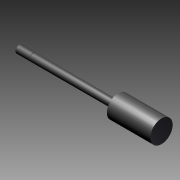
# Autodesk Inventor part: 0420_rod
Saved by Autodesk Inventor 2012 (Build 160160000, 160)
## iProperties
Category: PARTsolutions
Company: BIMBA
Created: 2013-01-19
Part Number: 0420_rod
Material: Default
Catalog Web Link: www.cadenas.de
Description: Standard Air Cylinder_rod-Original Line - Standard Air Cylinders
Vendor: BIMBA
Document SubType Name: Modeling
Designer: William
Manufacturer: BIMBA
Density: 1 g/cm^3
Mass: 13.5965 g
Surface Area: 45.5733 cm^2
Volume: 13.5965 cm^3
PSOL_IDENT_0: {\\10.0.0.242\data_v9\23d-libs\bimba\bimba\bimba_imperial\bimba_full_line\original_line_cylinders\st
PSOL_IDENT_1: andard_air_cylinders\rod.prj},270 {VTYP=3D},{NB=0420_rod},{LINA=0420_rod},{NN=Standard Air Cylinder_
PSOL_IDENT_2: rod},{DATE=11.09.2012 07:37:40},{GEOMDATE=06.09.2012 09:06:00},{VERSION=},{LINEID=50},{LINESUBID=-1}
PSOL_IDENT_3: ,{WBVAR=STROKE,ACTING,MNT,DER,NR,BM,CO,M,EE,EEL,K,Q,Y,F,G,T,B,H,SER,SR,NT,W,E,HL,ST,STP,PRC,PB,COLOR
PSOL_IDENT_4: 1}  {NB=0420_rod},{LINA=0420_rod},{KT=DUMMY},{PN=042},{DASH=},{BORE=0.75000000},{BOREPN=04},{STROKE=
PSOL_IDENT_5: 2.000},{STROKEALG=[0.001:50/0.001]},{STROKE1=2.000},{ACTING=},{ACTINGALG= '' , 'Single Acting' , 'R'
PSOL_IDENT_6: , 'Reverse Single Acting' , 'D' , 'Double Acting' },{ACTINGPN=},{MNT=},{MNTALG= '' , 'Front Nose Mo
PSOL_IDENT_7: unting' , 'P' , 'Rear Pivot Mounting' , 'BF' , 'Front Block Mounting' , 'BR' , 'Rear Block Mounting
PSOL_IDENT_8: for Vertical Positioning' , 'BFT' , 'Front Block Trunnion Mounting' , 'BRT' , 'Rear Block Trunnion M
PSOL_IDENT_9: ounting' , 'A' , 'Double End Mounting with Brackets and Adjustable Stroke' , 'AP' , 'Rear Pivot Moun
PSOL_IDENT_10: ting with Adjustable Stroke' },{TYPE=},{MNTPN=},{DER=},{DERALG= '' , 'N/A' },{NR=},{NRALG= '' , 'Sta
PSOL_IDENT_11: ndard' , 'NR' , 'Non-rotating - Hexagon Rod' },{NRPN=},{BM=},{BMALG= '' , 'Without Built-in Midget 3
PSOL_IDENT_12: -Way Solenoid Operated Valve' , 'LS' , 'With Built-in Midget 3-Way Solenoid Operated Valve' },{BMPN=
PSOL_IDENT_13: },{CO=},{COALG= '' , 'N/A' },{M=},{MALG= '', 'Without Magnet', 'M', 'With Magnet' },{EE=},{EEL=0},{E
PSOL_IDENT_14: EMAX=10},{EEALG= '', 'Without Extra Extension', 'EE', 'With Extra Extension' },{EELALG=0},{EEPN=},{E
PSOL_IDENT_15: EPN1=0.000},{K=},{KALG= '' , 'N/A' },{KPN=},{Q=},{QALG= '' , 'Without Side Ported Rear Head' , 'Q' ,
PSOL_IDENT_16: 'With Side Ported Rear Head' },{QPN=},{Y=},{YALG= '' , 'N/A' },{YPN=},{F=},{FALG= '', 'Standard', '
PSOL_IDENT_17: F', 'Molycoated Body' },{FPN=},{G=},{GPN=},{T=},{TALG= '' , 'Standard' , 'N' , 'Low Temperature' , '
PSOL_IDENT_18: V' , 'High Temperature' },{NPN=},{VPN=},{B=},{BALG= '', 'Without Bumper' , 'B' , 'With Bumper' },{BP
PSOL_IDENT_19: N=},{H=},{HALG= '', 'Standard', 'H', 'With Heavy Springs' },{HPN=},{SER=},{SERALG= '' , 'N/A' },{SR=
PSOL_IDENT_20: C},{SRALG= 'C' , 'Carbon Steel Rod' , 'SR' , '303 Stainless Steel Rod' , '' , '303 Stainless Steel R
PSOL_IDENT_21: od1' },{SRPN=},{SRCON=1},{NT=},{NTPN=},{W=},{WALG= '' , 'N/A' },{WPN=},{E=},{EALG= '' , 'Without Spe
PSOL_IDENT_22: cial Lube and Seals' , 'E' , 'With Special Lube and Seals' },{EPN=},{HL=},{HLALG= '' , 'N/A' },{ST=}
PSOL_IDENT_23: ,{STALG= '' , 'Without Switch Track' , 'T' , 'With Switch Track' },{STP=},{STPALG= '' , 'N/A' },{STP
PSOL_IDENT_24: N=},{PRC=},{PRCALG= '' , 'Without Piston Rod Clevis' , 'D-166-1' , 'With Piston Rod Clevis' },{PRCPN
PSOL_IDENT_25: =},{PB=},{PBALG= '' , 'Without Pivot Bracket' , 'D-167' , 'With Pivot Bracket' },{PBPN=},{TLEN=3.946
PSOL_IDENT_26: 0},{TEXT=0.233333},{SPACE=0.133333},{FRAC=5.5700},{RGCON=},{RGDACCON=},{RHCON=},{RHCONON=1},{RHACCON
PSOL_IDENT_27: =},{FNUTCON=1},{RNUTCON=0},{FNUTPN=D-98},{RNUTPN=},{FNUTTRANS=0.0000},{RNUTTRANS=0.0000},{VHOLECON=2
PSOL_IDENT_28: },{A1=0.8750},{A1N=0.8750},{A1P=1.5940},{A1B=1.5940},{A4=0.3130},{A4N=0.3130},{A4P=0.2525},{A5=0.030
PSOL_IDENT_29: 0},{A1H=0.531},{A1NH=0.5310},{A1PH=1.5940},{A1BH=1.0940},{A1SH=1.2190},{A2H=0.2190},{A2NH=0.2190},{L
PSOL_IDENT_30: ENGTH=1.5000},{LENGTH1=1.5000},{LENGTH2=3.0300},{MUL=3.3800},{MUL11=3.3800},{MUL22=5.3800},{MUL33=3.
PSOL_IDENT_31: 3800},{MUL2=1.6900},{MUL211=1.6900},{MUL222=2.6900},{MUL233=1.6900},{SSS=4.0000},{RGLEN=0.5920},{RHL
PSOL_IDENT_32: EN=0.3420},{SSS1=3.0000},{A13=1.3120},{THDLEN1=0.5000},{THD1=0.2500},{TAB=UNF},{THDLEN=0.5000},{THD=
PSOL_IDENT_33: 0.2500},{OD=0.7615},{RODL=4.8490},{PL=1.4740},{RODDIA=0.2500},{HEX=0.2500},{RODTRANS=0.0000},{G1=0.1
PSOL_IDENT_34: 250},{ON=0},{G5=0.6250},{DERLEN=3.3750},{THOLE=0.0000},{WF=0.2200},{BADD=0.0000},{MADD=0.0000},{NVAD
PSOL_IDENT_35: D=0.000},{JRADD=0.00000},{COLOR=0.00,0.00,0.00,0.00},{GROOVE=1},{HOL=0},{D7=0.2520},{H1=1.1175},{D1=
PSOL_IDENT_36: 0.8050},{D1RH=0.8050},{D1P=0.8325},{D1B=0.8625},{D1N=0.8050},{D1NRH=0.8050},{D1BRH=0.8325},{D1PRH=0.
PSOL_IDENT_37: 8625},{BOZO=0},{HADD=0.000},{COLOR1=0},{DEFL=0.0000},{HEXL=0.0000},{SSADD=0.0000},{WFL=0.0000},{MOVE
PSOL_IDENT_38: =0.0000}
CNS_NT: Standard
CNS_NB: 0420_rod
CNS_NBSYN: $PN.$COLOR1._rod
CNS_LINA: 0420_rod
CNS_PN: 042
CNS_BORE: 0.75000000
CNS_BOREPN: 04
CNS_STROKE: 2.000
CNS_STROKEALG: [0.001:50/0.001]
CNS_STROKE1: 2.000
CNS_ACTING: Single Acting
CNS_ACTINGALG: '' , 'Single Acting' , 'R' , 'Reverse Single Acting' , 'D' , 'Double Acting'
CNS_MNT: Front Nose Mounting
CNS_MNTALG: '' , 'Front Nose Mounting' , 'P' , 'Rear Pivot Mounting' , 'BF' , 'Front Block Mounting' , 'BR' , 'Rear Block Mounting for Vertical Positioning' , 'BFT' , 'Front Block Trunnion Mounting' , 'BRT' , 'Rear Block Trunnion Mounting' , 'A' , 'Double End Mounting with Brackets and Adjustable Stroke' , 'AP' , 'Rear Pivot Mounting with Adjustable Stroke'
CNS_DER: N/A
CNS_DERALG: '' , 'N/A'
CNS_NR: Standard
CNS_NRALG: '' , 'Standard' , 'NR' , 'Non-rotating - Hexagon Rod'
CNS_BM: Without Built-in Midget 3-Way Solenoid Operated Valve
CNS_BMALG: '' , 'Without Built-in Midget 3-Way Solenoid Operated Valve' , 'LS' , 'With Built-in Midget 3-Way Solenoid Operated Valve'
CNS_CO: N/A
CNS_COALG: '' , 'N/A'
CNS_M: Without Magnet
CNS_MALG: '', 'Without Magnet', 'M', 'With Magnet'
CNS_EE: Without Extra Extension
CNS_EEL: 0
CNS_EEMAX: 10
CNS_EEALG: '', 'Without Extra Extension', 'EE', 'With Extra Extension'
CNS_EELALG: 0
CNS_EEPN1: 0.000
CNS_K: N/A
CNS_KALG: '' , 'N/A'
CNS_Q: Without Side Ported Rear Head
CNS_QALG: '' , 'Without Side Ported Rear Head' , 'Q' , 'With Side Ported Rear Head'
CNS_Y: N/A
CNS_YALG: '' , 'N/A'
CNS_F: Standard
CNS_FALG: '', 'Standard', 'F', 'Molycoated Body'
CNS_G: Without Magnalube Lubrication
CNS_T: Standard
CNS_TALG: '' , 'Standard' , 'N' , 'Low Temperature' , 'V' , 'High Temperature'
CNS_B: Without Bumper
CNS_BALG: '', 'Without Bumper' , 'B' , 'With Bumper'
CNS_H: Standard
CNS_HALG: '', 'Standard', 'H', 'With Heavy Springs'
CNS_SER: N/A
CNS_SERALG: '' , 'N/A'
CNS_SR: Carbon Steel Rod
CNS_SRALG: 'C' , 'Carbon Steel Rod' , 'SR' , '303 Stainless Steel Rod' , '' , '303 Stainless Steel Rod1'
CNS_SRCON: 1
CNS_W: N/A
CNS_WALG: '' , 'N/A'
CNS_E: Without Special Lube and Seals
CNS_EALG: '' , 'Without Special Lube and Seals' , 'E' , 'With Special Lube and Seals'
CNS_HL: N/A
CNS_HLALG: '' , 'N/A'
CNS_ST: Without Switch Track
CNS_STALG: '' , 'Without Switch Track' , 'T' , 'With Switch Track'
CNS_STP: N/A
CNS_STPALG: '' , 'N/A'
CNS_PRC: Without Piston Rod Clevis
CNS_PRCALG: '' , 'Without Piston Rod Clevis' , 'D-166-1' , 'With Piston Rod Clevis'
CNS_PB: Without Pivot Bracket
CNS_PBALG: '' , 'Without Pivot Bracket' , 'D-167' , 'With Pivot Bracket'
CNS_TLEN: 3.9460
CNS_TEXT: 0.233
CNS_SPACE: 0.133
CNS_FRAC: 5.5700
CNS_RHCONON: 1
CNS_FNUTCON: 1
CNS_RNUTCON: 0
CNS_FNUTPN: D-98
CNS_FNUTTRANS: 0.0000
CNS_RNUTTRANS: 0.0000
CNS_VHOLECON: 2
CNS_A1: 0.8750
CNS_A1N: 0.8750
CNS_A1P: 1.5940
CNS_A1B: 1.5940
CNS_A4: 0.3130
CNS_A4N: 0.3130
CNS_A4P: 0.2525
CNS_A5: 0.0300
CNS_A1H: 0.531
CNS_A1NH: 0.5310
CNS_A1PH: 1.5940
CNS_A1BH: 1.0940
CNS_A1SH: 1.2190
CNS_A2H: 0.2190
CNS_A2NH: 0.2190
CNS_LENGTH: 1.5000
CNS_LENGTH1: 1.5000
CNS_LENGTH2: 3.0300
CNS_MUL: 3.3800
CNS_MUL11: 3.3800
CNS_MUL22: 5.3800
CNS_MUL33: 3.3800
CNS_MUL2: 1.6900
CNS_MUL211: 1.6900
CNS_MUL222: 2.6900
CNS_MUL233: 1.6900
CNS_SSS: 4.0000
CNS_RGLEN: 0.5920
CNS_RHLEN: 0.3420
CNS_SSS1: 3.0000
CNS_A13: 1.3120
CNS_THDLEN1: 0.5000
CNS_THD1: 0.2500
CNS_TAB: UNF
CNS_THDLEN: 0.5000
CNS_THD: 0.2500
CNS_OD: 0.7615
CNS_RODL: 4.8490
CNS_PL: 1.4740
CNS_RODDIA: 0.2500
CNS_HEX: 0.2500
CNS_RODTRANS: 0.0000
CNS_G1: 0.1250
CNS_ON: 0
CNS_G5: 0.6250
CNS_DERLEN: 3.3750
CNS_THOLE: 0.0000
CNS_WF: 0.2200
CNS_BADD: 0.0000
CNS_MADD: 0.0000
CNS_NVADD: 0.000
CNS_JRADD: 0.00000
CNS_COLOR: 0.00,0.00,0.00,0.00
CNS_GROOVE: 1
CNS_HOL: 0
CNS_D7: 0.2520
CNS_H1: 1.1175
CNS_D1: 0.8050
CNS_D1RH: 0.8050
CNS_D1P: 0.8325
CNS_D1B: 0.8625
CNS_D1N: 0.8050
CNS_D1NRH: 0.8050
CNS_D1BRH: 0.8325
CNS_D1PRH: 0.8625
CNS_BOZO: 0
CNS_HADD: 0.000
CNS_COLOR1: 0
CNS_DEFL: 0.0000
CNS_HEXL: 0.0000
CNS_SSADD: 0.0000
CNS_WFL: 0.0000
CNS_MOVE: 0.0000
SUPPLIER: BIMBA
ARTICLENO: 0420_rod
BOMINFO: 0420_rod
CREATOR: CADENAS GmbH
Title: 0420_rod
Author: Cadenas PARTsolutions
Comments: Original Line - Standard Air Cylinders
Autodesk Inventor part; units mm, degrees
sketch "Sketch_1" plane through (0, 0, 0) normal (0, 0, 1) x (1, 0, 0)
  line L0 (110.4646, 0) -> (0, 0)
  line L1 (0, 0) -> (0, 3.175)
  line L2 (0, 3.175) -> (73.025, 3.175)
  line L3 (73.025, 3.175) -> (73.025, 9.6203)
  line L4 (73.025, 9.6203) -> (110.4646, 9.6203)
  line L5 (110.4646, 9.6203) -> (110.4646, 0)
  line L6 (110.4646, 0) -> (0, 0)
  constraints: 14 end point
revolve "Revolution1" add sketch "Sketch_1" angle 360 about axis through (110.4646, 0, 0) along (1, 0, 0)
sketch "Sketch_3" plane through (0, 0, 0) normal (0, 0, 1) x (1, 0, 0)
  line L0 (0, 0) -> (-12.7, 0)
  line L1 (-12.7, 0) -> (-12.7, 2.634)
  line L2 (-12.7, 2.634) -> (-12.159, 3.175)
  line L3 (-12.159, 3.175) -> (0, 3.175)
  line L4 (0, 3.175) -> (0, 0)
  line L5 (0, 0) -> (-12.7, 0)
  constraints: 12 end point
revolve "Revolution2" add sketch "Sketch_3" angle 360 about axis through (0, 0, 0) along (1, 0, 0)
sketch "Sketch_30" plane through (0, 0, 0) normal (0, 0, 1) x (1, 0, 0)
  line L0 (0, 0) -> (-0.254, 0)
  line L1 (-0.254, 3.429) -> (-0.254, 2.921)
  line L2 (-0.254, 2.921) -> (0, 2.921)
  line L3 (0, 2.921) -> (0, 3.429)
  line L4 (0, 3.429) -> (-0.254, 3.429)
  constraints: 10 end point
revolve "Revolution3" cut sketch "Sketch_30" angle 360 about axis through (0, 0, 0) along (1, 0, 0)
ref_plane "rod_cp_XY" through (0, 0, 0) normal (1, 0, 0) x (0, 0, -1)
ref_plane "rod_cp_YZ" through (0, 0, 0) normal (0, 0, -1) x (0, 1, 0)
ref_plane "rod_cp_ZX" through (0, 0, 0) normal (0, 1, 0) x (1, 0, 0)
ref_plane "to_rod_clevis_XY" through (-12.7, 0, 0) normal (1, 0, 0) x (0, 0, -1)
ref_plane "to_rod_clevis_YZ" through (-12.7, 0, 0) normal (0, 0, -1) x (0, 1, 0)
ref_plane "to_rod_clevis_ZX" through (-12.7, 0, 0) normal (0, 1, 0) x (1, 0, 0)
ref_plane "rl2_XY" through (0, 0, 0) normal (1, 0, 0) x (0, 0, -1)
ref_plane "rl2_YZ" through (0, 0, 0) normal (0, 0, -1) x (0, 1, 0)
ref_plane "rl2_ZX" through (0, 0, 0) normal (0, 1, 0) x (1, 0, 0)
ref_plane "rl1_XY" through (-12.7, 0, 0) normal (1, 0, 0) x (0, 0, -1)
ref_plane "rl1_YZ" through (-12.7, 0, 0) normal (0, 0, -1) x (0, 1, 0)
ref_plane "rl1_ZX" through (-12.7, 0, 0) normal (0, 1, 0) x (1, 0, 0)
ref_plane "thd1_XY" through (-12.7, 3.175, 0) normal (1, 0, 0) x (0, 0, -1)
ref_plane "thd1_YZ" through (-12.7, 3.175, 0) normal (0, 0, -1) x (0, 1, 0)
ref_plane "thd1_ZX" through (-12.7, 3.175, 0) normal (0, 1, 0) x (1, 0, 0)
ref_plane "thd2_XY" through (-12.7, -3.175, 0) normal (1, 0, 0) x (0, 0, -1)
ref_plane "thd2_YZ" through (-12.7, -3.175, 0) normal (0, 0, -1) x (0, 1, 0)
ref_plane "thd2_ZX" through (-12.7, -3.175, 0) normal (0, 1, 0) x (1, 0, 0)
ref_plane "dia1_XY" through (0, 3.175, 0) normal (1, 0, 0) x (0, 0, -1)
ref_plane "dia1_YZ" through (0, 3.175, 0) normal (0, 0, -1) x (0, 1, 0)
ref_plane "dia1_ZX" through (0, 3.175, 0) normal (0, 1, 0) x (1, 0, 0)
ref_plane "dia2_XY" through (0, -3.175, 0) normal (1, 0, 0) x (0, 0, -1)
ref_plane "dia2_YZ" through (0, -3.175, 0) normal (0, 0, -1) x (0, 1, 0)
ref_plane "dia2_ZX" through (0, -3.175, 0) normal (0, 1, 0) x (1, 0, 0)
ref_plane "dia12_XY" through (0, 0, 10.2235) normal (1, 0, 0) x (0, 0, -1)
ref_plane "dia12_YZ" through (0, 0, 10.2235) normal (0, 0, -1) x (0, 1, 0)
ref_plane "dia12_ZX" through (0, 0, 10.2235) normal (0, 1, 0) x (1, 0, 0)
ref_plane "dia22_XY" through (0, 0, -10.2235) normal (1, 0, 0) x (0, 0, -1)
ref_plane "dia22_YZ" through (0, 0, -10.2235) normal (0, 0, -1) x (0, 1, 0)
ref_plane "dia22_ZX" through (0, 0, -10.2235) normal (0, 1, 0) x (1, 0, 0)
body "Solid1"
